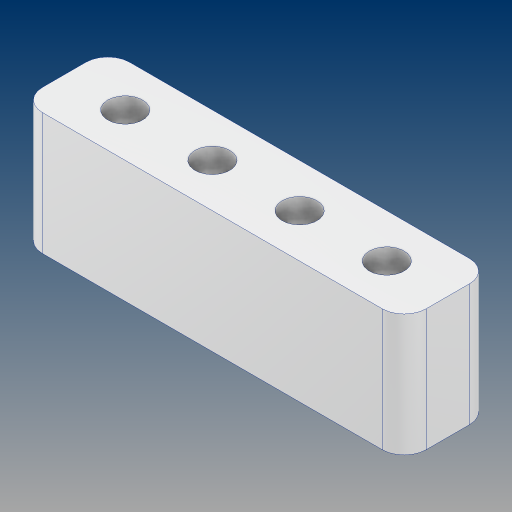
# Autodesk Inventor part: ELEV_023_BILLET2
Saved by Autodesk Inventor 2024.3 (Build 283343000, 343)
## iProperties
Created: 2024-11-28
Part Number: ELEV_023_BILLET2
Material: Aluminum 6061
Document SubType Name: Modeling
Designer: Kenji
Density: 2.7 g/cm^3
Appearance: Aluminum - Flat
Author: Kenji
Autodesk Inventor part; units mm, degrees
ref_plane "YZ Plane" through (0, 0, 0) normal (1, 0, 0) x (0, 1, 0)
ref_plane "XZ Plane" through (0, 0, 0) normal (0, 1, 0) x (-1, 0, 0)
ref_plane "XY Plane" through (0, 0, 0) normal (0, 0, 1) x (1, 0, 0)
sketch "Sketch1" plane through (0, 0, 0) normal (0, 1, 0) x (-1, 0, 0)
  line L0 (3.175, 0) -> (52.705, 0)
  line L1 (55.88, -3.175) -> (55.88, -9.525)
  line L2 (52.705, -12.7) -> (3.175, -12.7)
  line L3 (0, -9.525) -> (0, -3.175)
  circle A0 centre (46.99, -6.35) radius 2.54
  circle A1 centre (34.29, -6.35) radius 2.54
  circle A2 centre (21.59, -6.35) radius 2.54
  circle A3 centre (8.89, -6.35) radius 2.54
  line L4 (46.99, -6.35) -> (8.89, -6.35) construction
  arc A4 (52.705, -12.7) -> (55.88, -9.525) centre (52.705, -9.525) ccw
  arc A5 (55.88, -3.175) -> (52.705, 0) centre (52.705, -3.175) ccw
  arc A6 (3.175, 0) -> (0, -3.175) centre (3.175, -3.175) ccw
  arc A7 (0, -9.525) -> (3.175, -12.7) centre (3.175, -9.525) ccw
  point P0 (0, 0)
  dimension "d0" = 12.7
  dimension "d1" = 55.88
  dimension "d2" = 5.08
  dimension "d3" = 12.7
  dimension "d4" = 12.7
  dimension "d5" = 12.7
  dimension "d6" = 6.35
  dimension "d7" = 8.89
  dimension "d8" = 3.175
  constraints: 10 end point, 8 centre point, 8 point on circle, 8 tangent, 6 equal radius, 4 point on line, 2 parallel, 2 perpendicular, 1 horizontal
  measures "d0" distance between parallel lines of L2 L0
  measures "d1" distance between parallel lines of L3 L1
  measures "d2" diameter of A0
  measures "d3" distance of A1.centre L4.start
  measures "d4" distance of A2.centre A1.centre
  measures "d5" distance of L4.end A2.centre
  measures "d6" distance between parallel lines of L2 L4
  measures "d7" distance from line of L1 L4.start
  measures "d8" radius of A4
extrude "Extrusion1" add sketch "Sketch1" along normal blind 17.78
body "Solid1"
